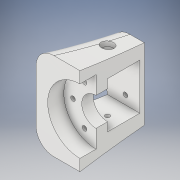
# Autodesk Inventor part: AA016
Saved by Autodesk Inventor 2017 SP1 (Build 210196100, 196)
## iProperties
Created: 2017-09-29
Part Number: AA016
Material: ABS Plastic
Document SubType Name: Modeling
Designer: Zach
Density: 1.06 g/cm^3
Appearance: CR White
Author: Zach
Autodesk Inventor part; units mm, degrees
ref_plane "YZ Plane" through (0, 0, 0) normal (1, 0, 0) x (0, 1, 0)
ref_plane "XY Plane" through (0, 0, 0) normal (0, 0, 1) x (1, 0, 0)
sketch "Sketch1" plane through (0, 0, 0) normal (0, 0, 1) x (1, 0, 0)
  line L0 (0, 0) -> (70, 0)
  line L1 (70, 0) -> (70, 77.5)
  line L2 (70, 77.5) -> (0, 77.5)
  line L3 (0, 77.5) -> (0, 0)
  dimension "d0" = 70
  dimension "d1" = 77.5
  constraints: 8 end point, 2 parallel, 1 horizontal, 1 perpendicular
  measures "d0" distance of L2.end L1.end
  measures "d1" distance of L1.end L0.end
extrude "Extrusion1" add sketch "Sketch1" along normal blind 70
sketch "Sketch3" plane through (0, 0, 70) normal (0, 0, 1) x (1, 0, 0)
  line L0 (0, 0) -> (70, 0) projected
  line L1 (70, 77.5) -> (0, 77.5) projected
  line L2 (70, 0) -> (35, 0)
  line L3 (35, 0) -> (35, 77.5)
  line L4 (35, 77.5) -> (70, 77.5)
  line L5 (70, 77.5) -> (70, 0)
  constraints: 8 end point, 2 parallel, 1 horizontal, 1 midpoint, 1 perpendicular
extrude "Extrusion3" cut sketch "Sketch3" against normal through all
sketch "Sketch4" plane through (0, 77.5, 70) normal (0, 1, 0) x (1, 0, 0)
  line L0 (0, 70) -> (0, 0) projected
  line L1 (0, 0) -> (-12.5, 0)
  line L2 (35, 70) -> (0, 70) projected
  arc A0 (-12.5, 0) -> (0, 70) centre (-1137.8005, 237.0626) ccw
  line L3 (-12.5, -10) -> (35, -10) construction
  dimension "d9" = 1150
  dimension "d54" = 47.5
  dimension "d55" = 10
  constraints: 4 end point, 2 horizontal, 2 point on circle, 2 vertical alignment, 1 centre point
  measures "d9" radius of A0
  measures "d54" distance of L3.start L3.end
  measures "d55" distance between parallel lines of L1 L3
extrude "Extrusion4" add sketch "Sketch4" against normal blind 77.5
sketch "Sketch5" plane through (35, 0, 70) normal (1, 0, 0) x (0, 0, -1)
  line L0 (0, 77.5) -> (0, 86.25)
  line L1 (0, 0) -> (0, -8.75)
  line L2 (0, 0) -> (0, 77.5) projected
  line L3 (70, 77.5) -> (70, 0) projected
  arc A0 (0, 86.25) -> (70, 77.5) centre (177.5728, 1222.4577) ccw
  arc A1 (70, 0) -> (0, -8.75) centre (177.5728, -1144.9577) ccw
  line L4 (0, 77.5) -> (70, 77.5) projected
  line L5 (70, 0) -> (0, 0) projected
  line L6 (-10, 86.25) -> (-10, -8.75) construction
  point P0 (-10, 38.75)
  point P1 (0, 38.75)
  dimension "d14" = 1150
  dimension "d15" = 1150
  dimension "d52" = 10
  dimension "d53" = 95
  constraints: 6 end point, 4 point on circle, 3 horizontal alignment, 3 vertical, 2 centre point, 2 midpoint
  measures "d14" radius of A0
  measures "d15" radius of A1
  measures "d52" distance between parallel lines of L2 L6
  measures "d53" distance of L6.start L6.end
extrude "Extrusion5" add sketch "Sketch5" against normal blind 55 contours L0 A0 L4 | L5 A1 L1
sketch "Sketch6" plane through (-20, 0, 0) normal (0, 1, 0) x (1, 0, 0)
  line L0 (20, 0) -> (0, 0) projected
  line L1 (0, -70) -> (0, 0) projected
  arc A0 (7.5, -70) -> (20, 0) centre (-1117.8005, 167.0626) ccw projected
  line L2 (7.5, -70) -> (0, -70) projected
extrude "Extrusion6" cut sketch "Sketch6" along normal through all both and the other way through all
fillet "Fillet3" radius 19.35 2 edges at (-5.7463, 81.368, 35.3063) (-5.7463, -3.868, 35.3063)
sketch "Sketch8" plane through (0, 0, 70) normal (0, 0, 1) x (1, 0, 0)
  line L0 (35, 86.25) -> (35, -8.75) projected
  line L1 (35, 77.5) -> (35, 0) projected
  circle A0 centre (35, 38.75) radius 35
  point P0 (0, 0)
  dimension "d23" = 70
  constraints: 1 centre point, 1 midpoint
  measures "d23" diameter of A0
extrude "Extrusion7" cut sketch "Sketch8" against normal blind 17.5
sketch "Sketch9" plane through (0, 0, 52.5) normal (0, 0, 1) x (1, 0, 0)
  line L0 (35, 73.75) -> (35, 3.75) projected
  circle A0 centre (35, 38.75) radius 15.5
  point P0 (0, 0)
  dimension "d26" = 31
  constraints: 1 centre point, 1 midpoint
  measures "d26" diameter of A0
extrude "Extrusion8" cut sketch "Sketch9" against normal blind 20
sketch "Sketch15" plane through (0, 0, 70) normal (0, 0, 1) x (1, 0, 0)
  circle A0 centre (10, 38.75) radius 2.5
  circle A1 centre (22.5, 17.0994) radius 2.5
  circle A2 centre (47.5, 17.0994) radius 2.5
  circle A3 centre (60, 38.75) radius 2.5
  circle A4 centre (47.5, 60.4006) radius 2.5
  circle A5 centre (22.5, 60.4006) radius 2.5
  arc A6 (35, 54.25) -> (35, 23.25) centre (35, 38.75) ccw projected
  point P0 (0, 0)
  dimension "d43" = 5
  dimension "d44" = 25
  dimension "d47" = 360
  constraints: 6 centre point, 1 coincident, 1 horizontal alignment, 13 other
  measures "d43" diameter of A0
  measures "d44" distance of point (35, 38.75) A0.centre
extrude "Extrusion13" cut sketch "Sketch15" against normal blind 25
sketch "Sketch17" plane through (35, 0, 0) normal (1, 0, 0) x (0, 0, -1)
  line L0 (-5, 13.75) -> (-40, 13.75)
  line L1 (-40, 13.75) -> (-40, 63.75)
  line L2 (-40, 63.75) -> (-5, 63.75)
  line L3 (-5, 63.75) -> (-5, 13.75)
  line L4 (0, 77.5) -> (0, 0) projected
  point P0 (-5, 38.75)
  point P1 (0, 38.75)
  dimension "d62" = 35
  dimension "d63" = 50
  dimension "d77" = 5
  constraints: 8 end point, 2 midpoint, 2 parallel, 1 horizontal, 1 horizontal alignment, 1 perpendicular
  measures "d62" distance of L1.end L2.end
  measures "d63" distance of L0.end L1.end
  measures "d77" distance between parallel lines of L4 L3
extrude "Extrusion15" cut sketch "Sketch17" against normal through all
sketch "Sketch18" plane through (35, 13.75, 40) normal (0, 1, 0) x (1, 0, 0)
  circle A0 centre (-15, 15) radius 2.5
  line L0 (0, -5) -> (0, 35)
  point P0 (-35, -5)
  point P1 (0, 0)
  point P2 (0, 15)
  dimension "d67" = 5
  dimension "d68" = 15
  constraints: 2 end point, 1 centre point, 1 horizontal alignment, 1 midpoint
  measures "d67" diameter of A0
  measures "d68" distance of point (0, 15) A0.centre
extrude "Extrusion16" cut sketch "Sketch18" along normal through all both and the other way through all
ref_plane "Work Plane1" through (35, 86.25, 70) normal (0, 1, 0) x (-1, 0, 0)
sketch "Sketch19" plane through (35, 86.25, 70) normal (0, 1, 0) x (-1, 0, 0)
  spline S0 degree 8 poles (12.5, -45) (12.5, -45.3028) (12.5419, -45.5982) (12.6221, -45.8795) (12.7361, -46.1415) (12.8782, -46.3795) (13.0421, -46.5905) (13.2208, -46.7727) (13.5844, -47.0735) (13.7727, -47.1977) (13.9687, -47.2997) (14.17, -47.3803) (14.3751, -47.4403) (14.5826, -47.4801) (14.7912, -47.5) (15.2606, -47.5) (15.521, -47.469) (15.7792, -47.4069) (16.0327, -47.3133) (16.2789, -47.1867) (16.5137, -47.0256) (16.732, -46.8284) (17.0926, -46.3926) (17.2469, -46.1571) (17.3764, -45.8907) (17.4709, -45.5997) (17.524, -45.2928) (17.5325, -44.9802) (17.4969, -44.6723) (17.3726, -44.1881) (17.3067, -44.0023) (17.2242, -43.8227) (17.1258, -43.6509) (17.0123, -43.4888) (16.8849, -43.3376) (16.7448, -43.1989) (16.4271, -42.936) (16.2471, -42.8148) (16.0554, -42.7116) (15.8541, -42.6276) (15.6455, -42.564) (15.432, -42.5213) (15.216, -42.5) (14.7912, -42.5) (14.5825, -42.5199) (14.3751, -42.5598) (14.17, -42.6197) (13.9686, -42.7004) (13.7727, -42.8024) (13.5844, -42.9265) (13.2209, -43.2272) (13.0422, -43.4095) (12.8782, -43.6205) (12.736, -43.8586) (12.6221, -44.1205) (12.5419, -44.4019) (12.5, -44.6973) (12.5, -45) knots 0 0 0 0 0 0 0 0 0 0.142624 0.142624 0.142624 0.142624 0.142624 0.142624 0.142624 0.279362 0.279362 0.279362 0.279362 0.279362 0.279362 0.279362 0.450047 0.450047 0.450047 0.450047 0.450047 0.450047 0.450047 0.596156 0.596156 0.596156 0.596156 0.596156 0.596156 0.596156 0.690678 0.690678 0.690678 0.690678 0.690678 0.690678 0.690678 0.794655 0.794655 0.794655 0.794655 0.794655 0.794655 0.794655 0.895176 0.895176 0.895176 0.895176 0.895176 0.895176 0.895176 1 1 1 1 1 1 1 1 1 projected
  circle A0 centre (15, -45) radius 2.5 projected
  circle A1 centre (15, -45) radius 6.5
  point P0 (35, -70)
  dimension "d71" = 13
  constraints: 1 centre point, 1 coincident, 1 vertical alignment, 1 other
  measures "d71" diameter of A1
extrude "Extrusion17" cut sketch "Sketch19" against normal blind 12
ref_plane "Work Plane2" through (35, -8.75, 70) normal (0, 1, 0) x (-1, 0, 0)
sketch "Sketch20" plane through (35, -8.75, 70) normal (0, 1, 0) x (-1, 0, 0)
  spline S0 degree 8 poles (12.5, -45) (12.5, -45.3028) (12.5419, -45.5982) (12.6221, -45.8795) (12.7361, -46.1415) (12.8782, -46.3795) (13.0421, -46.5905) (13.2208, -46.7727) (13.5844, -47.0735) (13.7727, -47.1977) (13.9687, -47.2997) (14.17, -47.3803) (14.3751, -47.4403) (14.5826, -47.4801) (14.7912, -47.5) (15.2606, -47.5) (15.521, -47.469) (15.7792, -47.4069) (16.0327, -47.3133) (16.2789, -47.1867) (16.5137, -47.0256) (16.732, -46.8284) (17.0926, -46.3926) (17.2469, -46.1571) (17.3764, -45.8907) (17.4709, -45.5997) (17.524, -45.2928) (17.5325, -44.9802) (17.4969, -44.6723) (17.3726, -44.1881) (17.3067, -44.0023) (17.2242, -43.8227) (17.1258, -43.6509) (17.0123, -43.4888) (16.8849, -43.3376) (16.7448, -43.1989) (16.4271, -42.936) (16.2471, -42.8148) (16.0554, -42.7116) (15.8541, -42.6276) (15.6455, -42.564) (15.432, -42.5213) (15.216, -42.5) (14.7912, -42.5) (14.5825, -42.5199) (14.3751, -42.5598) (14.17, -42.6197) (13.9686, -42.7004) (13.7727, -42.8024) (13.5844, -42.9265) (13.2209, -43.2272) (13.0422, -43.4095) (12.8782, -43.6205) (12.736, -43.8586) (12.6221, -44.1205) (12.5419, -44.4019) (12.5, -44.6973) (12.5, -45) knots 0 0 0 0 0 0 0 0 0 0.142624 0.142624 0.142624 0.142624 0.142624 0.142624 0.142624 0.279362 0.279362 0.279362 0.279362 0.279362 0.279362 0.279362 0.450047 0.450047 0.450047 0.450047 0.450047 0.450047 0.450047 0.596156 0.596156 0.596156 0.596156 0.596156 0.596156 0.596156 0.690678 0.690678 0.690678 0.690678 0.690678 0.690678 0.690678 0.794655 0.794655 0.794655 0.794655 0.794655 0.794655 0.794655 0.895176 0.895176 0.895176 0.895176 0.895176 0.895176 0.895176 1 1 1 1 1 1 1 1 1 projected
  circle A0 centre (15, -45) radius 6.5
  circle A1 centre (15, -45) radius 2.5 projected
  point P0 (35, -70)
  dimension "d74" = 13
  constraints: 1 centre point, 1 vertical alignment, 2 other
  measures "d74" diameter of A0
extrude "Extrusion18" cut sketch "Sketch20" along normal blind 12
sketch "Sketch21" plane through (0, 0, 0) normal (0, 0, -1) x (-1, 0, 0)
  circle A0 centre (-19.5, 54.25) radius 2.5
  circle A1 centre (-19.5, 23.25) radius 2.5
  line L0 (-35, 77.5) -> (-35, 0) projected
  line L1 (-19.5, 54.25) -> (-19.5, 23.25) construction
  point P0 (0, 0)
  point P1 (-35, 38.75)
  point P2 (-19.5, 38.75)
  dimension "d78" = 5
  dimension "d79" = 5
  dimension "d80" = 31
  dimension "d81" = 15.5
  constraints: 2 centre point, 2 end point, 2 midpoint, 1 horizontal alignment, 1 vertical
  measures "d78" diameter of A0
  measures "d79" diameter of A1
  measures "d80" distance of L1.start L1.end
  measures "d81" distance between parallel lines of L0 L1
extrude "Extrusion19" cut sketch "Sketch21" against normal blind 10
body "Solid1"
